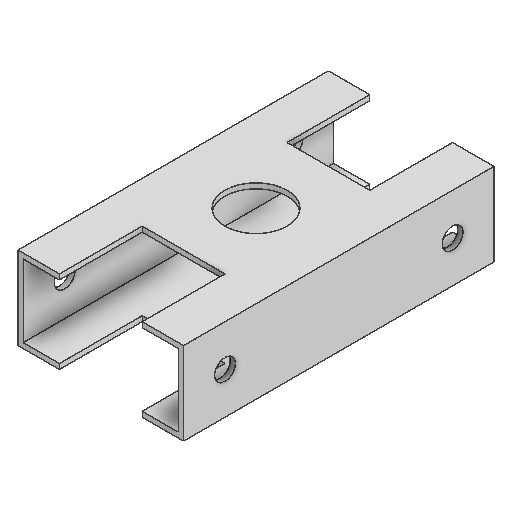
# Autodesk Inventor part: Diff Top Bar
Saved by Autodesk Inventor 2025.2 (Build 292293000, 293)
## iProperties
Created: 2025-02-20
Part Number: Diff Top Bar
Material: Generic
Document SubType Name: Modeling
Designer: Jakeg
Density: 1 g/cm^3
Appearance: Default
Author: Jakeg
Autodesk Inventor part; units mm, degrees
ref_plane "YZ Plane" through (0, 0, 0) normal (1, 0, 0) x (0, 1, 0)
ref_plane "XZ Plane" through (0, 0, 0) normal (0, 1, 0) x (-1, 0, 0)
ref_plane "XY Plane" through (0, 0, 0) normal (0, 0, 1) x (1, 0, 0)
sketch "Sketch1" plane through (0, 0, 0) normal (0, 0, 1) x (1, 0, 0)
  line L0 (-15.6216, 9.2219) -> (35.1784, 9.2219)
  line L1 (35.1784, 9.2219) -> (35.1784, -16.1781)
  line L2 (35.1784, -16.1781) -> (-15.6216, -16.1781)
  line L3 (-15.6216, -16.1781) -> (-15.6216, 9.2219)
  line L4 (-14.0341, 7.6344) -> (33.5909, 7.6344)
  line L5 (33.5909, 7.6344) -> (33.5909, -14.5906)
  line L6 (33.5909, -14.5906) -> (-14.0341, -14.5906)
  line L7 (-14.0341, -14.5906) -> (-14.0341, 7.6344)
  point P0 (0, 0)
  dimension "d0" = 50.8
  dimension "d1" = 25.4
  dimension "d2" = 1.5875
  dimension "d3" = 1.5875
  dimension "d4" = 1.5875
  dimension "d5" = 1.5875
  constraints: 16 end point, 4 parallel, 2 horizontal, 2 perpendicular
  measures "d0" distance of L0.start L0.end
  measures "d1" distance of L0.end L1.end
  measures "d2" distance between parallel lines of L3 L7
  measures "d3" distance between parallel lines of L1 L5
  measures "d4" distance between parallel lines of L2 L6
  measures "d5" distance between parallel lines of L0 L4
extrude "Extrusion1" add sketch "Sketch1" along normal blind 95.25
sketch "Sketch2" plane through (-15.6216, 9.2219, 0) normal (0, 1, 0) x (1, 0, 0)
  circle A0 centre (25.4, -47.625) radius 9.525
  line L0 (0, 0) -> (0, -95.25) projected
  line L1 (50.8, 0) -> (0, 0) projected
  line L2 (12.7, 0) -> (38.1, 0)
  line L3 (38.1, 0) -> (38.1, -25.4)
  line L4 (38.1, -25.4) -> (12.7, -25.4)
  line L5 (12.7, -25.4) -> (12.7, 0)
  line L6 (1.5875, -95.25) -> (49.2125, -95.25) projected
  line L7 (12.7, -95.25) -> (38.1, -95.25)
  line L8 (38.1, -95.25) -> (38.1, -69.85)
  line L9 (38.1, -69.85) -> (12.7, -69.85)
  line L10 (12.7, -69.85) -> (12.7, -95.25)
  point P0 (15.6216, 0)
  point P1 (25.4, -25.4)
  dimension "d8" = 19.05
  dimension "d9" = 25.4
  dimension "d10" = 47.625
  dimension "d13" = 25.4
  dimension "d14" = 25.4
  dimension "d15" = 25.4
  dimension "d16" = 25.4
  dimension "d25" = 95.25
  constraints: 16 end point, 4 parallel, 2 horizontal, 2 perpendicular, 2 point on line, 1 centre point, 1 midpoint
  measures "d8" diameter of A0
  measures "d9" distance from line of L0 A0.centre
  measures "d10" distance from line of L1 A0.centre
  measures "d13" distance of L3.end L4.end
  measures "d14" distance of L2.end L3.end
  measures "d15" distance from line of L0 point (25.4, -25.4)
  measures "d16" distance of L8.end L7.end
  measures "d25" distance between parallel lines of L6 L1
extrude "Extrusion2" cut sketch "Sketch2" against normal blind 116.84
sketch "Sketch3" plane through (35.1784, -16.1781, 0) normal (1, 0, 0) x (0, 0, -1)
  circle A0 centre (-12.7, 12.7) radius 3.175
  line L0 (0, 25.4) -> (-95.25, 25.4) projected
  circle A1 centre (-82.55, 12.7) radius 3.175
  line L1 (-95.25, 0) -> (-95.25, 25.4) projected
  point P0 (0, 16.1781)
  dimension "d17" = 6.35
  dimension "d18" = 12.7
  dimension "d19" = 12.7
  dimension "d20" = 6.35
  dimension "d21" = 12.7
  dimension "d22" = 12.7
  constraints: 2 centre point
  measures "d17" diameter of A0
  measures "d18" distance from line of L0 A0.centre
  measures "d19" horizontal distance of point (0, 16.178) A0.centre
  measures "d20" diameter of A1
  measures "d21" distance from line of L0 A1.centre
  measures "d22" distance from line of L1 A1.centre
extrude "Extrusion3" cut sketch "Sketch3" against normal through all
equation "\"d3\" = d2"
equation "\"d4\" = d2"
equation "\"d5\" = d2"
equation "\"d10\" = 0.5 * d25"
body "Solid1"
